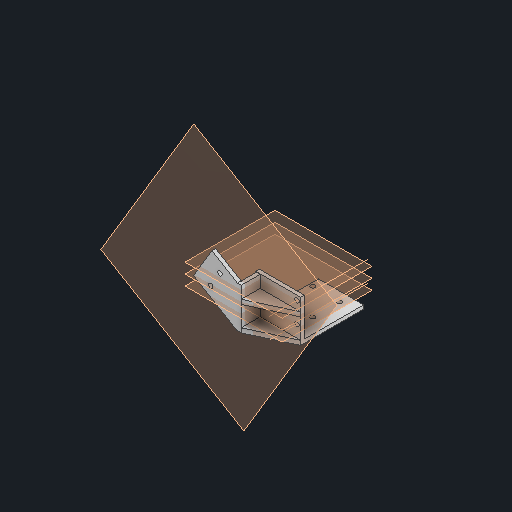
# Autodesk Inventor part: counter_sensor_holders
Saved by Autodesk Inventor 2024 (Build 280153000, 153)
## iProperties
Created: 2026-03-30
Part Number: counter_sensor_holders
Material: Generic
Document SubType Name: Modeling
Designer: schar
Density: 1 g/cm^3
Appearance: Default
Author: schar
Autodesk Inventor part; units mm, degrees
ref_plane "YZ Plane" through (0, 0, 0) normal (1, 0, 0) x (0, 1, 0)
ref_plane "XZ Plane" through (0, 0, 0) normal (0, 1, 0) x (-1, 0, 0)
ref_plane "XY Plane" through (0, 0, 0) normal (0, 0, 1) x (1, 0, 0)
sketch "Sketch1" plane through (0, 0, 0) normal (0, 0, 1) x (1, 0, 0)
  line L0 (-18.9826, -15.7) -> (4.0174, -15.7) projected
  line L1 (11.5, 10) -> (11.5, -10) projected
  line L2 (11.5, -10) -> (-11.5, -10) projected
  line L3 (-11.5, -10) -> (-11.5, 10) projected
  line L4 (-11.5, 10) -> (11.5, 10) projected
  line L5 (-18.9826, -15.7) -> (-18.9826, -14) projected
  line L6 (-18.9826, -15.7) -> (-18.9826, -18.2)
  line L7 (-18.9826, -18.2) -> (11.5, -18.2)
  line L8 (11.5, -18.2) -> (11.5, 10)
  line L9 (11.5, 10) -> (-18.9826, 10)
  line L10 (-18.9826, 10) -> (-18.9826, -18.2)
  point P0 (0, 0)
  dimension "d0" = 2.5
  constraints: 10 end point, 2 parallel, 1 horizontal, 1 perpendicular, 1 vertical
  measures "d0" distance of L0.start L6.end
extrude "Extrusion1" add sketch "Sketch1" along normal blind 2.5
sketch "Sketch2" plane through (0, 0, 0) normal (0, 0, -1) x (-1, 0, 0)
  line L0 (18.9826, 10) -> (18.9826, -18.2) projected
  line L1 (-11.5, -18.2) -> (-11.5, 10) projected
  line L2 (18.9826, -18.2) -> (-11.5, -18.2)
  line L3 (-11.5, -18.2) -> (-11.5, -15.7)
  line L4 (-11.5, -15.7) -> (18.9826, -15.7)
  line L5 (18.9826, -15.7) -> (18.9826, -18.2)
  point P0 (0, 0)
  dimension "d3" = 2.5
  constraints: 8 end point, 2 parallel, 1 horizontal, 1 perpendicular, 1 point on line
  measures "d3" distance of L2.end L3.end
extrude "Extrusion2" add sketch "Sketch2" along normal blind 40
sketch "Sketch4" plane through (-18.9826, -15.7, 0) normal (0, 1, 0) x (1, 0, 0)
  line L0 (23, 13.2181) -> (23, 36.2181) projected
  line L1 (23, 36.2181) -> (0, 36.2181) projected
  line L2 (0, 36.2181) -> (0, 13.2181) projected
  line L3 (0, 13.2181) -> (23, 13.2181) projected
  circle A0 centre (20.5, 15.7181) radius 1.5 projected
  circle A1 centre (20.5, 33.7181) radius 1.5 projected
  circle A2 centre (2.5, 33.7181) radius 1.5 projected
  circle A3 centre (2.5, 15.7181) radius 1.5 projected
  point P0 (18.9826, 0)
extrude "Extrusion3" cut sketch "Sketch4" against normal blind 40 contours A0 | A1 | A2 | A3
sketch "Sketch5" plane through (0, 0, 0) normal (0, 0, -1) x (-1, 0, 0)
  line L0 (9.8803, 8.3507) -> (9.8803, -8.3507) projected
  line L1 (9.8803, -8.3507) -> (5.0848, -8.3507) projected
  line L2 (5.0848, -8.3507) -> (5.0848, 8.3507) projected
  line L3 (5.0848, 8.3507) -> (9.8803, 8.3507) projected
  line L4 (-11.5, -10) -> (11.5, -10) projected
  line L5 (11.5, -10) -> (11.5, 10) projected
  line L6 (11.5, 10) -> (-11.5, 10) projected
  line L7 (-11.5, 10) -> (-11.5, -10) projected
  circle A0 centre (-9, -7) radius 1.5 projected
  circle A1 centre (-9, 7) radius 1.5 projected
  point P0 (0, 0)
extrude "Extrusion4" cut sketch "Sketch5" against normal blind 40 contours A0 | A1
ref_plane "Work Plane1" through (-2.2662, 39.9957, 12.7819) normal (0, 0, 1) x (-0.8579373, 0.5137544, 0)
sketch "Sketch6" plane through (-2.2662, 39.9957, 12.7819) normal (0, 0, 1) x (-0.8579373, 0.5137544, 0)
  line L0 (18.5, 0) -> (18.5, 93.5988) projected
  line L1 (-1.5, 0) -> (-1.5, 93.5988) projected
  line L2 (21.5, 18.6957) -> (-3.5, 18.6957) projected
  line L3 (-4.5, 75.0357) -> (21.5, 75.0357) projected
  line L4 (-15.5567, 58.5163) -> (-41.7088, 42.8558) projected
  line L5 (-15.5567, 58.5163) -> (18.5, 58.5163)
  line L6 (-27.221, 18.662) -> (-1.0688, 34.3225) projected
  line L7 (-1.0688, 34.3225) -> (18.5, 34.3225)
  line L8 (-1.5, 34.0643) -> (-15.9879, 58.2581)
  line L9 (-1.0688, 34.3225) -> (-1.6546, 34.3225)
  point P0 (-22.4922, 33.1495)
  constraints: 8 end point, 6 point on line, 2 perpendicular, 1 collinear, 1 horizontal
extrude "Extrusion5" add sketch "Sketch6" along normal blind 2.5 contours L7 L9 L1 L5 L0 | L1 L9 L8 L4 L5
sketch "Sketch7" plane through (-2.2662, 39.9957, 15.2819) normal (0, 0, 1) x (0.8579373, -0.5137544, 0)
  line L0 (15.5567, -58.5163) -> (41.7088, -42.8558) projected
  line L1 (15.9879, -58.2581) -> (18.1327, -56.9738)
  line L2 (1.6546, -34.3225) -> (-18.5, -34.3225) projected
  line L3 (1.6546, -34.3225) -> (5.6436, -31.9338)
  line L4 (15.9879, -58.2581) -> (1.6546, -34.3225) projected
  line L5 (18.1327, -56.9738) -> (1.8582, -29.7964)
  point P0 (22.4922, -33.1495)
  point P1 (3.7995, -33.0381)
  dimension "d12" = 2.5
  dimension "d13" = 2.5
  constraints: 6 end point, 2 perpendicular, 2 point on line
  measures "d12" distance of L1.start L1.end
  measures "d13" distance from line of L4 L1.end
extrude "Extrusion6" add sketch "Sketch7" against normal up to surface (12.7819 mm away)
sketch "Sketch8" plane through (-18.9826, -18.2, -40) normal (0, -1, 0) x (1, 0, 0)
  line L0 (3.0026, 55.2819) -> (3.0026, 42.5) projected
  line L1 (30.4826, 0) -> (30.4826, 42.5) projected
  line L2 (3.0026, 55.2819) -> (30.4826, 42.5)
  line L3 (30.4826, 42.5) -> (3.0026, 42.5)
  point P0 (18.9826, 40)
  constraints: 4 end point, 1 perpendicular
extrude "Extrusion7" add sketch "Sketch8" against normal blind 3
ref_plane "Work Plane4" through (9, 0, 0) normal (0, 1, 0) x (0, 0, 1)
ref_plane "Work Plane2" through (9, -7, 0) normal (0, 1, 0) x (0, 0, 1)
ref_plane "Work Plane3" through (9, 7, 2.5) normal (0, 1, 0) x (0, 0, -1)
sketch "Sketch9" plane through (9, 0, 0) normal (0, 1, 0) x (0, 0, 1)
  line L0 (-40, 2.5) -> (2.5, 2.5) projected
  line L1 (15.2819, -24.98) -> (15.2819, -27.48) projected
  line L2 (2.5, 2.5) -> (15.2819, -24.98)
  line L3 (15.2819, -24.98) -> (2.5, -24.98)
  line L4 (2.5, -24.98) -> (15.2819, -24.98)
  line L5 (2.5, 2.5) -> (2.5, -27.9826) projected
  line L6 (2.5, -24.98) -> (2.5, 2.5)
  point P0 (0, -9)
  constraints: 8 end point, 2 collinear, 1 perpendicular
extrude "Extrusion8" add sketch "Sketch9" along normal mid plane 3
sketch "Sketch10" plane through (-2.2662, 39.9957, 15.2819) normal (0, 0, 1) x (0.8579373, -0.5137544, 0)
  line L0 (-6.3751, 0) -> (-6.3751, -93.5988) projected
  line L1 (-10.4351, 0) -> (-10.4351, -93.5988) projected
  line L2 (-6.3751, -46.7994) -> (-10.4351, -46.7994)
  circle A0 centre (-8.4051, -46.7994) radius 1.5
  line L3 (1.6546, -34.3225) -> (-18.5, -34.3225) projected
  line L4 (-6.3751, -34.3225) -> (-6.3751, -46.7994)
  line L5 (-6.3751, -40.561) -> (-10.4351, -40.561)
  line L6 (-18.5, -58.5163) -> (15.5567, -58.5163) projected
  line L7 (-6.3751, -58.5163) -> (-6.3751, -46.7994)
  line L8 (-6.3751, -52.6579) -> (-10.4351, -52.6579)
  circle A1 centre (-8.4051, -52.6579) radius 1.5
  circle A2 centre (-8.4051, -40.561) radius 1.5
  point P0 (22.4922, -33.1495)
  dimension "d22" = 3
  dimension "d23" = 3
  dimension "d24" = 3
  constraints: 10 end point, 7 midpoint, 6 point on line, 3 centre point, 2 collinear, 2 perpendicular
  measures "d22" diameter of A0
  measures "d23" diameter of A1
  measures "d24" diameter of A2
extrude "Extrusion9" cut sketch "Sketch10" against normal blind 3 contours A2 L5 | L5 A2 | A1 L8 | L8 A1
body "Solid1"
